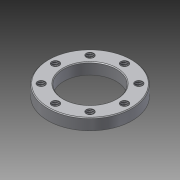
# Autodesk Inventor part: Rotary Pneumatic Cylinder Axis
Saved by Autodesk Inventor 2014 SP1 (Build 180222100, 222)
## iProperties
Created: 2013-12-16
Part Number: Rotary Pneumatic Cylinder Axis
Material: Aluminum 6061
Document SubType Name: Modeling
Designer: Moses
Density: 2.71 g/cm^3
Appearance: Aluminum - Flat
Mass: 55.7492 g
Surface Area: 91.7823 cm^2
Volume: 20.5717 cm^3
Author: Moses
Autodesk Inventor part; units mm, degrees
ref_plane "YZ Plane" through (0, 0, 0) normal (1, 0, 0) x (0, 1, 0)
ref_plane "XZ Plane" through (0, 0, 0) normal (0, 1, 0) x (-1, 0, 0)
ref_plane "XY Plane" through (0, 0, 0) normal (0, 0, 1) x (1, 0, 0)
sketch "Sketch1" plane through (0, 0, 0) normal (0, 1, 0) x (-1, 0, 0)
  circle A0 centre (0, 0) radius 35.56
  circle A1 centre (0, 0) radius 22.225
  line L0 (0, 0) -> (29.21, 0) construction
  circle A2 centre (29.21, 0) radius 3.175
  circle A3 centre (20.6546, 20.6546) radius 3.175
  circle A4 centre (0, 29.21) radius 3.175
  circle A5 centre (-20.6546, 20.6546) radius 3.175
  circle A6 centre (-29.21, 0) radius 3.175
  circle A7 centre (-20.6546, -20.6546) radius 3.175
  circle A8 centre (0, -29.21) radius 3.175
  circle A9 centre (20.6546, -20.6546) radius 3.175
  dimension "d0" = 71.12
  dimension "d1" = 44.45
  dimension "d2" = 29.21
  dimension "d3" = 6.35
  dimension "d6" = 360
  constraints: 10 centre point, 3 coincident, 2 end point, 1 horizontal, 17 other
  measures "d0" diameter of A0
  measures "d1" diameter of A1
  measures "d2" distance of L0.start L0.end
  measures "d3" diameter of A2
extrude "Extrusion1" add sketch "Sketch1" along normal blind 9.525
thread "Thread1" size "1/4-20 UNC" class "2B" standard "ANSI Unified Screw Threads" full length
thread "Thread2" size "1/4-20 UNC" class "2B" standard "ANSI Unified Screw Threads" full length
thread "Thread3" size "1/4-20 UNC" class "2B" standard "ANSI Unified Screw Threads" full length
thread "Thread4" size "1/4-20 UNC" class "2B" standard "ANSI Unified Screw Threads" full length
thread "Thread5" size "1/4-20 UNC" class "2B" standard "ANSI Unified Screw Threads" full length
thread "Thread6" size "1/4-20 UNC" class "2B" standard "ANSI Unified Screw Threads" full length
thread "Thread7" size "1/4-20 UNC" class "2B" standard "ANSI Unified Screw Threads" full length
thread "Thread8" size "1/4-20 UNC" class "2B" standard "ANSI Unified Screw Threads" full length
chamfer "Chamfer1" distance 0.635 angle 45 2 edges at (35.56, 9.525, 0) (22.225, 9.525, 0)
equation "\"d2\" = 0.5 * d0 - d3"
body "Solid1"
